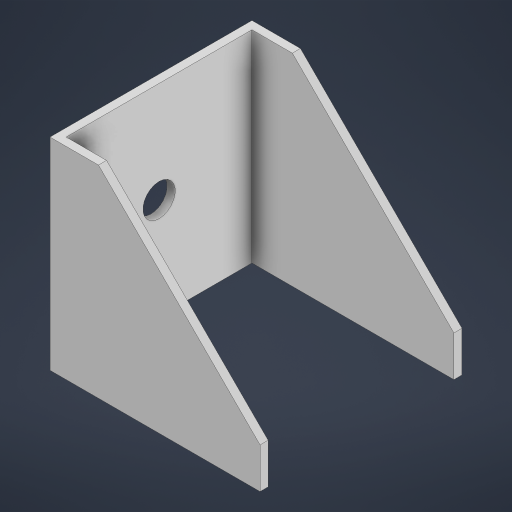
# Autodesk Inventor part: Tensioner_fix
Saved by Autodesk Inventor 2023 (Build 270158000, 158)
## iProperties
Created: 2023-11-08
Part Number: Tensioner_fix
Material: Generic
Document SubType Name: Modeling
Designer: Abhinav
Density: 1 g/cm^3
Appearance: Default
Author: Abhinav
Autodesk Inventor part; units mm, degrees
ref_plane "YZ Plane" through (0, 0, 0) normal (1, 0, 0) x (0, 1, 0)
ref_plane "XZ Plane" through (0, 0, 0) normal (0, 1, 0) x (-1, 0, 0)
ref_plane "XY Plane" through (0, 0, 0) normal (0, 0, 1) x (1, 0, 0)
sketch "Sketch1" plane through (0, 0, 0) normal (1, 0, 0) x (0, 1, 0)
  line L0 (25, 25) -> (-25, 25)
  line L1 (-25, 25) -> (-25, -25)
  line L2 (-25, -25) -> (25, -25)
  line L3 (25, -25) -> (25, 25)
  line L4 (25, 25) -> (-25, -25) construction
  line L5 (-25, 25) -> (25, -25) construction
  circle A0 centre (0, 0) radius 4
  dimension "d0" = 50
  dimension "d1" = 50
  dimension "d11" = 8
  constraints: 12 end point, 2 midpoint, 2 parallel, 1 centre point, 1 coincident, 1 horizontal, 1 perpendicular
  measures "d0" distance of L2.end L1.end
  measures "d1" distance of L1.end L0.end
  measures "d11" diameter of A0
extrude "Extrusion1" add sketch "Sketch1" along normal blind 2
sketch "Sketch2" plane through (0, -25, 25) normal (0, 0, 1) x (1, 0, 0)
  line L0 (2, 0) -> (52, 0)
  line L1 (52, 0) -> (52, 10)
  line L2 (2, 0) -> (2, 50) projected
  line L3 (2, 50) -> (12, 50)
  line L4 (12, 50) -> (52, 10)
  point P0 (0, 25)
  dimension "d4" = 50
  dimension "d5" = 10
  dimension "d6" = 10
  constraints: 8 end point, 2 horizontal, 1 perpendicular
  measures "d4" distance of L0.start L0.end
  measures "d5" distance of L0.end L1.end
  measures "d6" distance of L2.end L3.end
extrude "Extrusion2" add sketch "Sketch2" against normal blind 2
sketch "Sketch3" plane through (0, -25, -25) normal (0, 0, -1) x (-1, 0, 0)
  line L0 (-52, 0) -> (-2, 0) projected
  line L1 (-2, 50) -> (-2, 0) projected
  line L2 (-2, 50) -> (-12, 50) projected
  line L3 (-12, 50) -> (-52, 10) projected
  line L4 (-52, 10) -> (-52, 0) projected
  point P0 (0, 25)
extrude "Extrusion3" add sketch "Sketch3" against normal blind 2
body "Solid1"
